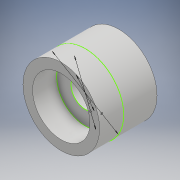
# Autodesk Inventor part: magnet_holder
Saved by Autodesk Inventor 2018 (Build 220112000, 112)
## iProperties
Created: 2017-06-18
Part Number: magnet_holder
Material: Ogólny
Document SubType Name: Modeling
Designer: Karol
Density: 1 g/cm^3
Appearance: Domyślna
Author: Karol
Autodesk Inventor part; units mm, degrees
ref_plane "YZ Plane" through (0, 0, 0) normal (1, 0, 0) x (0, 1, 0)
ref_plane "XZ Plane" through (0, 0, 0) normal (0, 1, 0) x (-1, 0, 0)
ref_plane "XY Plane" through (0, 0, 0) normal (0, 0, 1) x (1, 0, 0)
sketch "Sketch1" plane through (0, 0, 0) normal (0, 1, 0) x (-1, 0, 0)
  circle A0 centre (0, 0) radius 4
  circle A1 centre (0, 0) radius 3
  circle A2 centre (0, 0) radius 1.5
  dimension "d4" = 8
  dimension "d11" = 6
  dimension "d12" = 3
  constraints: 3 centre point, 3 coincident
  measures "d4" diameter of A0
  measures "d11" diameter of A1
  measures "d12" diameter of A2
extrude "Wyciągnięcie proste5" add sketch "Sketch1" against normal blind 2.5 contours A0
extrude "Wyciągnięcie proste6" add sketch "Sketch1" along normal blind 3.5 contours A0 | A1
